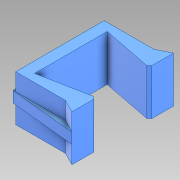
# Autodesk Inventor part: StraightRais-215
Saved by Autodesk Inventor 2021 (Build 250183000, 183)
## iProperties
Created: 2021-02-11
Part Number: StraightRais-215
Material: ABS プラスチック
Document SubType Name: Modeling
Designer: kumagai
Density: 1.06 g/cm^3
Appearance: 滑らか - 青
cp: 0.000 mm
ConnectorLength: 15.000 mm
RailWidth: 38.000 mm
JointFH: 9.500 mm
PrinterOffset: 0.000 mm
StraightLength: 215.000 mm
OuterWall: 2.000 mm
InnerWall: 2.400 mm
InsideWidth: 18.600 mm
RailHeight: 8.400 mm
RailDepth: 3.200 mm
JointMW1: 13.000 mm
JointMW2: 9.400 mm
JointMH: 9.000 mm
JointFW1: 13.300 mm
JointFW2: 9.600 mm
SupportGap: 0.200 mm
SupportRib: 0.500 mm
Author: kumagai
Autodesk Inventor part; units mm, degrees
ref_plane "YZ Plane" through (0, 0, 0) normal (1, 0, 0) x (0, 1, 0)
ref_plane "XZ Plane" through (0, 0, 0) normal (0, 1, 0) x (-1, 0, 0)
ref_plane "XY Plane" through (0, 0, 0) normal (0, 0, 1) x (1, 0, 0)
sketch "スケッチ1" plane through (0, 0, 0) normal (0, 1, 0) x (-1, 0, 0)
  line L0 (0, -13.02) -> (0, 13.02) projected
  line L1 (-2.4, 0) -> (14.4, 0) projected
  line L2 (0, -4.8) -> (9.5, -6.65)
  line L3 (9.5, -6.65) -> (9.5, 6.65)
  line L4 (9.5, 6.65) -> (0, 4.8)
  line L5 (0, -9.3) -> (0, -4.8)
  line L6 (0, 4.8) -> (0, 9.3)
  line L7 (2.4, -8.1) -> (11.5, -8.1)
  line L8 (11.5, -8.1) -> (11.5, 8.1)
  line L9 (11.5, 8.1) -> (2.4, 8.1)
  line L10 (2.4, -8.1) -> (0, -9.3)
  line L11 (2.4, 8.1) -> (0, 9.3)
  line L12 (12, -8.1) -> (12, 8.1)
  line L13 (12, 8.1) -> (0, 9.3)
  line L14 (12, -8.1) -> (0, -9.3)
  point P0 (0, 0)
  point P1 (0, 9.3)
  point P2 (0, -9.3)
  dimension "d3" = 13.3
  dimension "d5" = 9.6
  dimension "d14" = 2
  dimension "d63" = 1.2
  dimension "d64" = 18.6
  dimension "d65" = 12
  dimension "d74" = 18.6
  dimension "d75" = 1.2
  dimension "d93" = 9.5
  dimension "d94" = 2.4
  constraints: 26 end point, 2 collinear, 2 horizontal, 2 point on line, 2 vertical, 1 parallel, 1 symmetric about line, 3 other
  measures "d3" distance of L3.end L2.end
  measures "d5" distance of L4.end L2.start
  measures "d14" distance between parallel lines of L3 L8
  measures "d63" vertical distance of L10.end L7.start
  measures "d64" distance of L11.end L10.end
  measures "d65" distance between parallel lines of L12 L0
  measures "d74" distance of L5.start L6.end
  measures "d75" vertical distance of L12.end L6.end
  measures "d93" distance between parallel lines of L0 L3
  measures "d94" distance from line of L0 L7.start
extrude "押し出し2" add sketch "スケッチ1" along normal blind 3.2 and the other way blind 5.2 contours L0 L2 L3 L1 L8 L7 L10 | L0 L11 L9 L8 L1 L3 L4
extrude "押し出し1" add sketch "スケッチ1" against normal blind 2 contours L0 L2 L3 L1 L8 L7 L10 | L10 L7 L8 L1 L12 L14 | L1 L8 L9 L11 L13 L12 | L0 L11 L9 L8 L1 L3 L4
chamfer "面取り3" distance 0.5 angle 45 2 edges at (0, -1, 4.8) (0, -1, -4.8)
equation "\"rib\" = 0.5"
equation "\"gap\" = 0.2"
